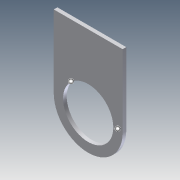
# Autodesk Inventor part: Blank Button Lable
Saved by Autodesk Inventor 2016 (Build 200138000, 138)
## iProperties
Created: 2005-06-20
Part Number: Blank Button Lable
Checked By: ~
Material: Generic
Document SubType Name: Modeling
Designer: BassBW
Manufacturer: Standard
Standards Organization: Custom
Density: 1 g/cm^3
Appearance: White
SCALE: 1:1
STOCK SIZE: SEE DWG
UNITS: ANSI
COMMODITY: MFG
Author: BassBW
Autodesk Inventor part; units mm, degrees
ref_plane "YZ Plane" through (0, 0, 0) normal (1, 0, 0) x (0, 1, 0)
ref_plane "XZ Plane" through (0, 0, 0) normal (0, 1, 0) x (-1, 0, 0)
ref_plane "XY Plane" through (0, 0, 0) normal (0, 0, 1) x (1, 0, 0)
sketch "Sketch1" plane through (0, 0, 0) normal (0, 0, 1) x (1, 0, 0)
  line L0 (30.1625, 0) -> (30.1625, 31.75)
  line L1 (30.1625, 31.75) -> (0, 31.75)
  line L2 (0, 31.75) -> (0, 0)
  arc A0 (0, 0) -> (30.1625, 0) centre (15.0813, 0) ccw
  dimension "d34" = 30.1625
  dimension "d35" = 31.75
  constraints: 6 end point, 2 point on circle, 2 tangent, 1 centre point, 1 horizontal, 1 parallel, 1 vertical
  measures "d34" distance of L0.end L1.end
  measures "d35" distance from line of A0.centre L1
extrude "Extrusion6" add sketch "Sketch1" along normal blind 1.5875
sketch "Sketch9" plane through (0, 0, 1.5875) normal (0, 0, 1) x (1, 0, 0)
  arc A0 (0, 0) -> (30.1625, 0) centre (15.0813, 0) ccw projected
  circle A1 centre (15.0813, 0) radius 11
  dimension "d38" = 22
  constraints: 1 centre point, 1 coincident
  measures "d38" diameter of A1
extrude "Extrusion7" cut sketch "Sketch9" against normal through all
body "Solid1"
